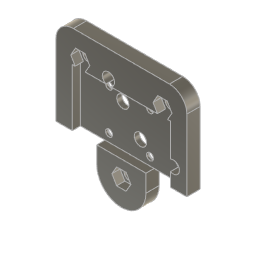
cr6 mgn12h adapter (Autodesk Fusion 360 design; units mm, degrees)
Autodesk Fusion 360 part; units mm, degrees
note: some values were not read from the file. Set by a fixed rule: which sketch regions a step uses.
sketch "Sketch1" plane through (0, 0, 0) normal (0, 1, 0) x (1, 0, 0)
  circle A0 centre (0, 0) radius 12
  line L0 (32, -52) -> (-32, -52)
  line L1 (-32, -52) -> (-32, -8.5)
  line L2 (-32, -8.5) -> (32, -8.5)
  line L3 (32, -8.5) -> (32, -52)
  line L4 (0, 0) -> (0, -52) construction
  line L5 (-12, 0) -> (-12, -8.5)
  line L6 (12, 0) -> (12, -8.5)
  dimension "d1" = 24
  dimension "d2" = 64
  dimension "d3" = 43.5
  dimension "d4" = 64
  constraint coincident A0.centre L4.start
  constraint horizontal L0
  constraint vertical L1
  constraint horizontal L2
  constraint vertical L3
  constraint midpoint L0 L4.end
  constraint vertical L4
  constraint coincident A0 L5.start
  constraint coincident L2 L5.end
  constraint coincident A0 L6.start
  constraint coincident L2 L6.end
  constraint tangent A0 L6
  constraint tangent A0 L5
  constraint vertical L5
  constraint vertical L6
  measures "d1" diameter of A0
  measures "d3" distance of L0 L2
  measures "d4" distance of L1 L3
extrude "Extrude1" add sketch "Sketch1" along normal blind 6.5
fillet "Fillet1" radius 8.5 2 edges at (-32, 3.25, 52) (32, 3.25, 52)
sketch "Sketch2" plane through (0, 0, 0) normal (0, -1, 0) x (1, 0, 0)
  line L0 (-12, 8.5) -> (-12, 0)
  arc A0 (-12, 0) -> (12, 0) centre (0, 0) ccw
  line L1 (12, 0) -> (12, 8.5)
  line L2 (12, 8.5) -> (32, 8.5)
  line L3 (32, 8.5) -> (32, 43.5)
  line L4 (23.5, 52) -> (-23.5, 52)
  line L5 (-32, 43.5) -> (-32, 8.5)
  line L6 (-32, 8.5) -> (-12, 8.5)
  line L7 (-32, 40.215) -> (32, 40.215) construction
  circle A1 centre (-20.1, 40.215) radius 2.5 construction
  circle A2 centre (0, 0) radius 2.5 construction
  circle A3 centre (20.1, 40.215) radius 2.5 construction
  line L8 (0, 0) -> (0, 48) construction
  line L9 (-17.7906, 36.215) -> (-15.4812, 40.215)
  line L10 (-15.4812, 40.215) -> (-17.7906, 44.215)
  line L11 (-17.7906, 44.215) -> (-22.4094, 44.215)
  line L12 (-22.4094, 44.215) -> (-24.7188, 40.215)
  line L13 (-24.7188, 40.215) -> (-22.4094, 36.215)
  line L14 (-22.4094, 36.215) -> (-17.7906, 36.215)
  line L15 (22.4094, 36.215) -> (24.7188, 40.215)
  line L16 (24.7188, 40.215) -> (22.4094, 44.215)
  line L17 (22.4094, 44.215) -> (17.7906, 44.215)
  line L18 (17.7906, 44.215) -> (15.4812, 40.215)
  line L19 (15.4812, 40.215) -> (17.7906, 36.215)
  line L20 (17.7906, 36.215) -> (22.4094, 36.215)
  line L21 (2.3094, -4) -> (4.6188, 0)
  line L22 (4.6188, 0) -> (2.3094, 4)
  line L23 (2.3094, 4) -> (-2.3094, 4)
  line L24 (-2.3094, 4) -> (-4.6188, 0)
  line L25 (-4.6188, 0) -> (-2.3094, -4)
  line L26 (-2.3094, -4) -> (2.3094, -4)
  arc A4 (32, 43.5) -> (23.5, 52) centre (23.5, 43.5) ccw
  arc A5 (-23.5, 52) -> (-32, 43.5) centre (-23.5, 43.5) ccw
  point P0 (-20.1, 40.215)
  point P1 (20.1, 40.215)
  dimension "d7" = 40.215
  dimension "d8" = 5
  dimension "d9" = 5
  dimension "d10" = 5
  dimension "d11" = 20.1
  dimension "d12" = 20.1
  dimension "d13" = 4
  dimension "d14" = 4
  dimension "d45" = 4
  constraint coincident L5 L7.start
  constraint coincident L3 L7.end
  constraint perpendicular L3 L7
  constraint coincident L7 P0
  constraint coincident A0.centre A2.centre
  constraint coincident L7 P1
  constraint perpendicular L7 L8
  constraint coincident P0 A1.centre
  constraint coincident P1 A3.centre
  constraint horizontal L26
  measures "d7" distance of A0.centre L7
  measures "d8" diameter of A1
  measures "d9" diameter of A2
  measures "d10" diameter of A3
  measures "d11" distance of P0 L8
  measures "d12" distance of P1 L8
  measures "d13" distance of P0 L14
  measures "d14" distance of A0.centre L26
  measures "d45" distance of P1 L20
hole "Hole1" at (-20.1, 0, 40.215) at (20.1, 0, 40.215) at (0, 0, 0) direction (0, 1, 0) diameter 5.5 depth 16 tip angle 118
sketch "Sketch3" plane through (0, 0, 0) normal (0, -1, 0) x (1, 0, 0)
  circle A0 centre (20.1, 40.215) radius 2.75
  circle A1 centre (-20.1, 40.215) radius 2.75
  circle A2 centre (0, 0) radius 2.75
  line L0 (-12, 8.5) -> (-12, 0)
  arc A3 (-12, 0) -> (12, 0) centre (0, 0) ccw
  line L1 (12, 0) -> (12, 8.5)
  line L2 (12, 8.5) -> (32, 8.5)
  line L3 (32, 8.5) -> (32, 43.5)
  line L4 (23.5, 52) -> (-23.5, 52)
  line L5 (-32, 43.5) -> (-32, 8.5)
  line L6 (-32, 8.5) -> (-12, 8.5)
  line L7 (0, 0) -> (0, 52) construction
  line L8 (32, 0) -> (-32, 0) construction
  circle A4 centre (5.32, 17.45) radius 3
  circle A5 centre (25.4, 17.815) radius 3
  circle A6 centre (-3.25, 29.2) radius 3
  circle A7 centre (-6.3, 39.25) radius 3
  arc A8 (32, 43.5) -> (23.5, 52) centre (23.5, 43.5) ccw
  arc A9 (-23.5, 52) -> (-32, 43.5) centre (-23.5, 43.5) ccw
  dimension "d18" = 6
  dimension "d19" = 17.45
  dimension "d20" = 5.32
  dimension "d21" = 6
  dimension "d22" = 25.4
  dimension "d23" = 17.815
  dimension "d24" = 6
  dimension "d25" = 6
  dimension "d26" = 6.3
  dimension "d27" = 3.25
  dimension "d28" = 39.25
  dimension "d29" = 29.2
  constraint coincident A2.centre A3.centre
  constraint midpoint L4 L7.end
  constraint perpendicular L3 L8
  measures "d18" diameter of A4
  measures "d19" distance of L8 A4.centre
  measures "d20" distance of L7 A4.centre
  measures "d21" diameter of A5
  measures "d22" distance of L7 A5.centre
  measures "d23" distance of L8 A5.centre
  measures "d24" diameter of A7
  measures "d25" diameter of A6
  measures "d26" distance of L7 A7.centre
  measures "d27" distance of L7 A6.centre
  measures "d28" distance of L8 A7.centre
  measures "d29" distance of L8 A6.centre
extrude "Extrude2" cut sketch "Sketch3" against normal through all contours A4 | A5 | A6 | A7
sketch "Sketch4" plane through (0, 0, 0) normal (0, -1, 0) x (1, 0, 0)
  circle A0 centre (5.32, 17.45) radius 3
  circle A1 centre (-3.25, 29.2) radius 3
  circle A2 centre (25.4, 17.815) radius 3
  circle A3 centre (-6.3, 39.25) radius 3
  circle A4 centre (20.1, 40.215) radius 2.75
  circle A5 centre (-20.1, 40.215) radius 2.75
  circle A6 centre (0, 0) radius 2.75
  line L0 (-12, 8.5) -> (-12, 0)
  arc A7 (-12, 0) -> (12, 0) centre (0, 0) ccw
  line L1 (12, 0) -> (12, 8.5)
  line L2 (12, 8.5) -> (32, 8.5)
  line L3 (32, 8.5) -> (32, 43.5)
  line L4 (23.5, 52) -> (-23.5, 52)
  line L5 (-32, 43.5) -> (-32, 8.5)
  line L6 (-32, 8.5) -> (-12, 8.5)
  line L7 (0, 56) -> (0, 0) construction
  line L8 (41, 0) -> (0, 0) construction
  line L9 (24, 8.5) -> (-24, 8.5)
  line L10 (-24, 8.5) -> (-24, 36.5)
  line L11 (-24, 36.5) -> (24, 36.5)
  line L12 (24, 36.5) -> (24, 8.5)
  line L13 (24, 8.5) -> (-24, 36.5) construction
  line L14 (-24, 8.5) -> (24, 36.5) construction
  line L15 (10, 32.5) -> (-10, 32.5) construction
  line L16 (-10, 32.5) -> (-10, 12.5) construction
  line L17 (-10, 12.5) -> (10, 12.5) construction
  line L18 (10, 12.5) -> (10, 32.5) construction
  line L19 (10, 32.5) -> (-10, 12.5) construction
  line L20 (-10, 32.5) -> (10, 12.5) construction
  arc A8 (32, 43.5) -> (23.5, 52) centre (23.5, 43.5) ccw
  arc A9 (-23.5, 52) -> (-32, 43.5) centre (-23.5, 43.5) ccw
  point P0 (0, 22.5)
  point P1 (0, 22.5)
  dimension "d31" = 48
  dimension "d32" = 28
  dimension "d33" = 20
  dimension "d34" = 20
  dimension "d35" = 8.5
  constraint coincident A6.centre A7.centre
  constraint horizontal L9
  constraint perpendicular L9 L10
  constraint parallel L9 L11
  constraint parallel L10 L12
  constraint coincident L13 P1
  constraint coincident L14 P1
  constraint coincident L7 P1
  constraint horizontal L15
  constraint perpendicular L15 L16
  constraint parallel L15 L17
  constraint parallel L16 L18
  constraint coincident L19 P1
  constraint coincident L20 P1
  constraint coincident P1 P0
  measures "d31" distance of L10.end L11.end
  measures "d32" distance of L9.end L10.end
  measures "d33" distance of L16.end L17.end
  measures "d34" distance of L15.end L16.end
  measures "d35" distance of L8 L9
extrude "Extrude3" cut sketch "Sketch4" against normal blind 4 contours A2 A3 L2 L6 L9 L10 L11 L12 | A3 L11 picked at (-6.5707, 36.454)
extrude "Extrude4" cut sketch "Sketch2" against normal blind 4 contours L9 L10 L11 L12 L13 L14 | L15 L16 L17 L18 L19 L20 | L21 L22 L23 L24 L25 L26
sketch "Sketch5" plane through (0, 6.5, 0) normal (0, 1, 0) x (-1, 0, 0)
  circle A0 centre (-5.32, 17.45) radius 3
  circle A1 centre (3.25, 29.2) radius 3
  circle A2 centre (-25.4, 17.815) radius 3
  circle A3 centre (6.3, 39.25) radius 3
  circle A4 centre (-20.1, 40.215) radius 2.75
  circle A5 centre (20.1, 40.215) radius 2.75
  circle A6 centre (0, 0) radius 2.75
  line L0 (12, 0) -> (12, 8.5)
  line L1 (12, 8.5) -> (32, 8.5)
  line L2 (32, 8.5) -> (32, 43.5)
  line L3 (23.5, 52) -> (-23.5, 52)
  line L4 (-32, 43.5) -> (-32, 8.5)
  line L5 (-32, 8.5) -> (-12, 8.5)
  line L6 (-12, 8.5) -> (-12, 0)
  arc A7 (-12, 0) -> (12, 0) centre (0, 0) ccw
  line L7 (-10, 32.5) -> (10, 32.5)
  line L8 (-10, 12.5) -> (-10, 32.5)
  line L9 (10, 32.5) -> (10, 12.5)
  line L10 (10, 12.5) -> (-10, 12.5)
  arc A8 (-23.5, 52) -> (-32, 43.5) centre (-23.5, 43.5) ccw
  arc A9 (32, 43.5) -> (23.5, 52) centre (23.5, 43.5) ccw
hole "Hole2" at (10, 6.5, 32.5) at (10, 6.5, 12.5) at (-10, 6.5, 12.5) at (-10, 6.5, 32.5) direction (0, -1, 0) diameter 3.4 depth 16 tip angle 118 countersink diameter 6.3 countersink angle 90
